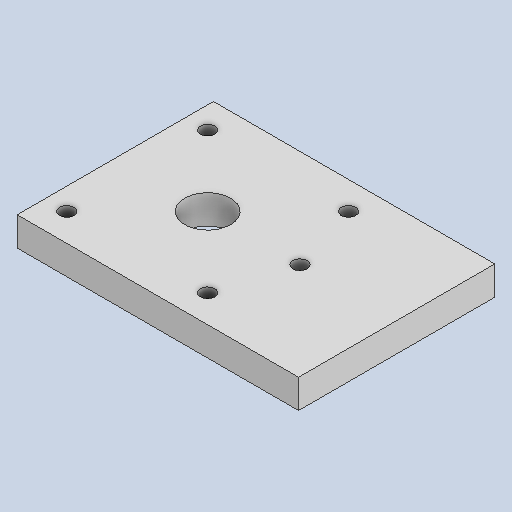
# Autodesk Inventor part: AR-BracketLeft2
Saved by Autodesk Inventor 2025.1 (Build 291241020, 241B)
## iProperties
Created: 2025-05-09
Part Number: AR-BracketLeft2
Material: Generic
Document SubType Name: Modeling
Designer: t205b
Density: 1 g/cm^3
Appearance: Default
Author: t205b
Autodesk Inventor part; units mm, degrees
ref_plane "YZ Plane" through (0, 0, 0) normal (1, 0, 0) x (0, 1, 0)
ref_plane "XZ Plane" through (0, 0, 0) normal (0, 1, 0) x (-1, 0, 0)
ref_plane "XY Plane" through (0, 0, 0) normal (0, 0, 1) x (1, 0, 0)
sketch "Sketch1" plane through (0, 0, 0) normal (0, 1, 0) x (-1, 0, 0)
  line L0 (0, 0) -> (61.9125, 0)
  line L1 (61.9125, 0) -> (61.9125, -43.18)
  line L2 (61.9125, -43.18) -> (0, -43.18)
  line L3 (0, -43.18) -> (0, 0)
  dimension "d0" = 61.9125
  dimension "d1" = 43.18
  constraints: 8 end point, 2 parallel, 1 horizontal, 1 perpendicular
  measures "d0" distance between parallel lines of L3 L1
  measures "d1" distance between parallel lines of L0 L2
extrude "Extrusion1" add sketch "Sketch1" along normal blind 6.35
sketch "Sketch2" plane through (0, 6.35, 0) normal (0, 1, 0) x (1, 0, 0)
  line L0 (-61.9125, 43.18) -> (-61.9125, 0)
  line L1 (-61.9125, 0) -> (0, 0)
  line L2 (0, 0) -> (0, 43.18)
  line L3 (-61.9125, 43.18) -> (0, 43.18)
  line L4 (-61.9125, 43.18) -> (-61.9125, 0) projected
  line L5 (0, 43.18) -> (-61.9125, 43.18) projected
  line L6 (-61.9125, 0) -> (0, 0) projected
  line L7 (0, 0) -> (0, 43.18) projected
  point P0 (-41.5925, 21.59)
  point P1 (-57.0925, 37.09)
  point P2 (-57.0925, 6.09)
  point P3 (-26.0925, 6.09)
  point P4 (-21.2725, 21.59)
  point P5 (-26.0925, 37.09)
  dimension "d4" = 6.09
  dimension "d5" = 4.82
  dimension "d6" = 6.09
  dimension "d7" = 4.82
  dimension "d8" = 6.09
  dimension "d9" = 26.0925
  dimension "d10" = 21.2725
  dimension "d11" = 21.59
  dimension "d12" = 6.09
  dimension "d13" = 26.0925
  dimension "d14" = 21.59
  dimension "d15" = 20.32
  constraints: 8 end point, 4 collinear
  measures "d4" distance from line of L1 point (-57.093, 6.09)
  measures "d5" distance from line of point (-57.093, 6.09) L0
  measures "d6" distance from line of point (-57.093, 37.09) L3
  measures "d7" distance from line of point (-57.093, 37.09) L0
  measures "d8" distance from line of point (-26.092, 37.09) L3
  measures "d9" distance from line of L2 point (-26.092, 37.09)
  measures "d10" distance from line of L2 point (-21.272, 21.59)
  measures "d11" distance from line of L1 point (-21.272, 21.59)
  measures "d12" distance from line of L1 point (-26.092, 6.09)
  measures "d13" distance from line of L2 point (-26.092, 6.09)
  measures "d14" distance from line of L1 point (-41.593, 21.59)
  measures "d15" distance from line of L0 point (-41.593, 21.59)
hole "Hole1" at (-57.0925, 6.35, -37.09) at (-57.0925, 6.35, -6.09) at (-26.0925, 6.35, -6.09) at (-26.0925, 6.35, -37.09) at (-21.2725, 6.35, -21.59) direction (0, -1, 0) diameter 3.175 depth 10.9728 tip angle 118
hole "Hole2" at (-41.5925, 6.35, -21.59) direction (0, -1, 0) diameter 10.1001 depth 10.9728 tip angle 118
sketch "Sketch3" plane through (-61.9125, 0, -43.18) normal (-1, 0, 0) x (0, 0, 1)
  line L0 (0, 0) -> (0, 6.35) projected
  line L1 (43.18, 0) -> (43.18, 6.35) projected
  line L2 (0, 6.35) -> (43.18, 6.35) projected
  point P0 (11.43, 3.175)
  point P1 (31.75, 3.175)
  dimension "d37" = 11.43
  dimension "d38" = 11.43
  dimension "d39" = 3.175
  constraints: 1 horizontal alignment
  measures "d37" distance from line of L0 point (11.43, 3.175)
  measures "d38" distance from line of L1 point (31.75, 3.175)
  measures "d39" distance from line of point (31.75, 3.175) L2
hole "Hole3" at (-61.9125, 3.175, -31.75) at (-61.9125, 3.175, -11.43) direction (1, 0, 0) diameter 2.6416 depth 12.7 tip angle 118 thread size "6-32 UNC" class "3B" standard "ANSI Unified Screw Threads"
body "Solid1"
